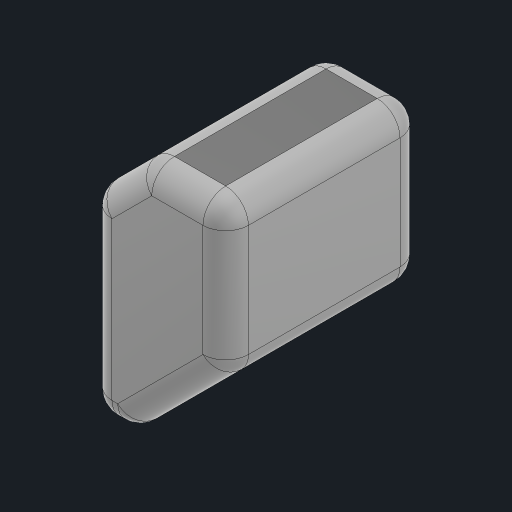
# Autodesk Inventor part: Ar620
Saved by Autodesk Inventor 2023.2 (Build 272271030, 271C)
## iProperties
Created: 2024-02-18
Part Number: Ar620
Material: ABS Plastic
Document SubType Name: Modeling
Designer: robpl
Density: 1.06 g/cm^3
Appearance: Smooth - Medium Gray
Mass: 7.42788 g
Surface Area: 47.0932 cm^2
Volume: 7.00743 cm^3
Author: robpl
Autodesk Inventor part; units mm, degrees
ref_plane "YZ Plane" through (0, 0, 0) normal (1, 0, 0) x (0, 1, 0)
ref_plane "XZ Plane" through (0, 0, 0) normal (0, 1, 0) x (-1, 0, 0)
ref_plane "XY Plane" through (0, 0, 0) normal (0, 0, 1) x (1, 0, 0)
sketch "Sketch1" plane through (0, 0, 0) normal (0, 0, 1) x (1, 0, 0)
  line L0 (0, 0) -> (-18, 0)
  line L1 (-18, 0) -> (-18, -32)
  line L2 (-18, -32) -> (0, -32)
  line L3 (0, -32) -> (0, 0)
  dimension "d0" = 18
  dimension "d1" = 32
  constraints: 8 end point, 2 parallel, 1 horizontal, 1 perpendicular
  measures "d0" distance of L2.end L1.end
  measures "d1" distance of L1.end L0.end
extrude "Extrusion1" add sketch "Sketch1" along normal mid plane 26
chamfer "Chamfer1" distance 7 angle 45 1 edges at (-18, 0, 0)
chamfer "Chamfer2" distance 13 angle 45 1 edges at (0, -32, 0)
fillet "Fillet1" radius 3 18 edges at (-18, -7, 0) (-11, 0, 0) (0, 0, 0) (0, -9.5, -13) (-5.5, 0, -13) (-14.5, -3.5, -13) (-18, -19.5, -13) (-15.5, -32, -13) (-18, -32, 0) (-15.5, -32, 13) (-18, -19.5, 13) (-14.5, -3.5, 13) (-5.5, 0, 13) (0, -9.5, 13) (0, -19, 0) (-6.5, -25.5, -13) (-13, -32, 0) (-6.5, -25.5, 13)
sketch "Sketch2" plane through (0, 0, 0) normal (0, 0, 1) x (1, 0, 0)
  line L0 (-15, -29) -> (-15, -8.2426) projected
  line L1 (-14.2426, -29) -> (-15, -29) projected
  line L2 (-3, -17.7574) -> (-14.2426, -29) projected
  line L3 (-3, -3) -> (-3, -17.7574) projected
  line L4 (-9.7574, -3) -> (-3, -3) projected
  line L5 (-15, -8.2426) -> (-9.7574, -3) projected
  point P0 (0, 0)
extrude "Extrusion2" cut sketch "Sketch2" along normal mid plane 20
body "Solid1"
